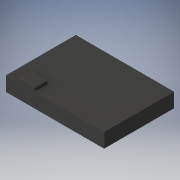
# Autodesk Inventor part: FONA
Saved by Autodesk Inventor 2018 (Build 220112000, 112)
## iProperties
Created: 2017-05-31
Part Number: FONA
Material: Acetal Resin, Black
Document SubType Name: Modeling
Designer: Rishi
Density: 1.425 g/cm^3
Appearance: Smooth - Black
Author: Rishi
Autodesk Inventor part; units mm, degrees
ref_plane "YZ Plane" through (0, 0, 0) normal (1, 0, 0) x (0, 1, 0)
ref_plane "XZ Plane" through (0, 0, 0) normal (0, 1, 0) x (-1, 0, 0)
ref_plane "XY Plane" through (0, 0, 0) normal (0, 0, 1) x (1, 0, 0)
sketch "Sketch1" plane through (0, 0, 0) normal (0, 1, 0) x (-1, 0, 0)
  line L0 (45, 32) -> (0, 32)
  line L1 (0, 32) -> (0, 0)
  line L2 (0, 0) -> (45, 0)
  line L3 (45, 0) -> (45, 32)
  dimension "d0" = 45
  dimension "d1" = 32
  constraints: 8 end point, 2 parallel, 1 horizontal, 1 perpendicular
  measures "d0" distance of L0.start L0.end
  measures "d1" distance of L2.end L0.start
extrude "Extrusion1" add sketch "Sketch1" along normal blind 6.55
sketch "Sketch2" plane through (0, 6.55, 0) normal (0, 1, 0) x (1, 0, 0)
  line L0 (-45, -32) -> (0, -32) projected
  line L1 (-40, -26) -> (-32, -26)
  line L2 (-32, -26) -> (-32, -32)
  line L3 (-32, -32) -> (-40, -32)
  line L4 (-40, -32) -> (-40, -26)
  line L5 (-45, 0) -> (-45, -32) projected
  point P0 (0, 0)
  dimension "d4" = 8
  dimension "d5" = 6
  dimension "d6" = 5
  constraints: 8 end point, 2 parallel, 1 horizontal, 1 perpendicular, 1 point on line
  measures "d4" distance of L1.start L1.end
  measures "d5" distance of L1.end L2.end
  measures "d6" distance between parallel lines of L5 L4
extrude "Extrusion2" add sketch "Sketch2" along normal blind 1.45
body "Solid1"
